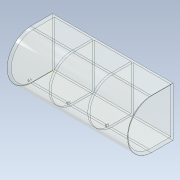
# Autodesk Inventor part: DeckelKoch_Better
Saved by Autodesk Inventor 2020 (Build 240168000, 168)
## iProperties
Created: 2022-02-02
Part Number: DeckelKoch_Better
Material: Glas
Document SubType Name: Modeling
Designer: Julian Uhl
Density: 2.18 g/cm^3
Appearance: Klar
Mass: 1224.67 g
Surface Area: 2271.98 cm^2
Volume: 561.774 cm^3
Author: Julian Uhl
Autodesk Inventor part; units mm, degrees
ref_plane "YZ Plane" through (0, 0, 0) normal (1, 0, 0) x (0, 1, 0)
ref_plane "XZ Plane" through (0, 0, 0) normal (0, 1, 0) x (-1, 0, 0)
ref_plane "XY Plane" through (0, 0, 0) normal (0, 0, 1) x (1, 0, 0)
sketch "Skizze1" plane through (0, 0, 0) normal (0, 0, 1) x (1, 0, 0)
  line L0 (-56, 0) -> (336, 0) projected
  line L1 (0, -23) -> (0, 138) projected
  line L2 (0, 0) -> (280, 0)
  line L3 (280, 0) -> (280, 115)
  line L4 (280, 115) -> (0, 115)
  line L5 (0, 115) -> (0, 0)
  line L6 (5, 5) -> (275, 5)
  line L7 (275, 5) -> (275, 110)
  line L8 (275, 110) -> (5, 110)
  line L9 (5, 110) -> (5, 5)
  dimension "d0" = 280
  dimension "d1" = 115
  dimension "d2" = 5
  dimension "d3" = 5
  dimension "d4" = 5
  dimension "d5" = 5
  constraints: 16 end point, 4 parallel, 2 horizontal, 2 perpendicular
  measures "d0" distance between parallel lines of L3 L5
  measures "d1" distance between parallel lines of L2 L4
  measures "d2" distance between parallel lines of L4 L8
  measures "d3" distance between parallel lines of L2 L6
  measures "d4" distance between parallel lines of L9 L5
  measures "d5" distance between parallel lines of L3 L7
extrude "Extrusion1" add sketch "Skizze1" along normal blind 50
sketch "Skizze3" plane through (280, 0, 0) normal (1, 0, 0) x (0, 0, -1)
  line L0 (-50, 115) -> (-50, 0) projected
  arc A0 (-50, 115) -> (-50, 0) centre (-47.5962, 57.5) ccw
  line L1 (-50, 5) -> (-50, 110) projected
  line L2 (0, 110) -> (-50, 110) projected
  arc A1 (-50, 110) -> (-50, 5) centre (-47.5962, 57.5) ccw
  point P0 (0, 0)
  dimension "d8" = 52.555
  constraints: 4 point on circle, 2 centre point, 1 coincident, 1 concentric
  measures "d8" radius of A1
extrude "Extrusion2" add sketch "Skizze3" against normal blind 275 contours L0 A1 A0
sketch "Skizze4" plane through (0, 115, 0) normal (0, 1, 0) x (1, 0, 0)
  line L0 (0, -50) -> (5, -50) projected
  line L1 (5, -50) -> (5, -105.1465) projected
  line L2 (0, -50) -> (5, -50)
  line L3 (5, -50) -> (5, -105.1465)
  line L4 (5, -105.1465) -> (0, -105.1465)
  line L5 (0, -105.1465) -> (0, -50)
  line L6 (5, -50) -> (275, -50) projected
  line L7 (280, -105.1465) -> (5, -105.1465) projected
  line L8 (275, -50) -> (280, -50)
  line L9 (280, -50) -> (280, -105.1465)
  line L10 (280, -105.1465) -> (275, -105.1465)
  line L11 (275, -105.1465) -> (275, -50)
  point P0 (0, 0)
  constraints: 16 end point, 4 parallel, 2 horizontal, 2 perpendicular, 1 point on line
extrude "Extrusion3" add sketch "Skizze4" against normal blind 115 contours L0 L1 L4 L5 | L8 L9 L7 L11
sketch "Skizze5" plane through (0, 0, 0) normal (-1, 0, 0) x (0, 0, 1)
  line L0 (50, 0) -> (105.1465, 0) projected
  arc A0 (105.1465, 57.5) -> (50, 115) centre (47.5962, 57.5) ccw projected
  line L1 (105.1465, 57.5) -> (105.1465, 0) projected
  arc A1 (50, 0) -> (50, 115) centre (47.5962, 57.5) ccw
  point P0 (0, 0)
  constraints: 3 point on circle, 1 centre point
extrude "Extrusion4" cut sketch "Skizze5" against normal blind 115
sketch "Skizze6" plane through (0, 0, 0) normal (-1, 0, 0) x (0, 0, 1)
  line L0 (105.1465, 115) -> (105.1465, 57.5) projected
  arc A0 (105.1465, 57.5) -> (50, 115) centre (47.5962, 57.5) ccw projected
  arc A1 (105.1465, 57.5) -> (50, 115) centre (47.5962, 57.5) ccw
  line L1 (50, 115) -> (105.1465, 115)
  line L2 (105.1465, 57.5) -> (105.1465, 115)
  point P0 (0, 0)
  constraints: 4 end point, 2 point on circle, 2 tangent, 1 centre point, 1 collinear, 1 horizontal
extrude "Extrusion5" cut sketch "Skizze6" against normal blind 115
sketch "Skizze7" plane through (280, 0, 0) normal (1, 0, 0) x (0, 0, -1)
  line L0 (0, 115) -> (-105.1465, 115) projected
  arc A0 (-105.1465, 57.5) -> (-50, 0) centre (-47.5962, 57.5) ccw projected
  arc A1 (-50, 115) -> (-105.1465, 57.5) centre (-47.5962, 57.5) ccw projected
  arc A2 (-52.5732, 115) -> (-50, 0) centre (-47.5081, 57.5845) ccw
  line L1 (-105.1465, 0) -> (-50, 0) projected
  line L2 (-50, 0) -> (-105.1465, 0)
  line L3 (-105.1465, 0) -> (-105.1465, 115)
  line L4 (-105.1465, 115) -> (-52.5732, 115)
  point P0 (0, 0)
  point P1 (-105.1465, 57.6691)
  constraints: 6 end point, 3 point on circle, 2 perpendicular, 1 centre point, 1 horizontal, 1 midpoint
extrude "Extrusion6" cut sketch "Skizze7" against normal blind 115
sketch "Skizze8" plane through (0, 0, 0) normal (0, 0, -1) x (-1, 0, 0)
  line L0 (-275, 5) -> (-5, 5) projected
  line L1 (-92.5, 5) -> (-92.5, 110)
  line L2 (-5, 110) -> (-275, 110) projected
  line L3 (-97.5, 5) -> (-97.5, 110)
  line L4 (-182.5, 5) -> (-182.5, 110)
  line L5 (-187.5, 5) -> (-187.5, 110)
  line L6 (0, 115) -> (0, 0) projected
  line L7 (-280, 0) -> (-280, 115) projected
  dimension "d20" = 5
  dimension "d22" = 5
  dimension "d23" = 92.5
  dimension "d24" = 92.5
  constraints: 8 end point, 8 point on line, 3 perpendicular, 1 vertical
  measures "d20" distance between parallel lines of L1 L3
  measures "d22" distance between parallel lines of L5 L4
  measures "d23" distance between parallel lines of L1 L6
  measures "d24" distance between parallel lines of L7 L5
extrude "Extrusion7" add sketch "Skizze8" against normal blind 115 contours L5 L2 L4 L0 | L3 L2 L1 L0
sketch "Skizze9" plane through (280, 0, 0) normal (1, 0, 0) x (0, 0, -1)
  arc A0 (-50, 115) -> (-50, 0) centre (-47.5962, 57.5) ccw projected
  arc A1 (-50, 115) -> (-50, 0) centre (-47.5962, 57.5) ccw
  line L0 (-50, 0) -> (-115, 0)
  line L1 (-71.1712, 5) -> (-115, 5) projected
  line L2 (-115, 0) -> (-115, 115)
  line L3 (-115, 5) -> (-115, 110) projected
  line L4 (-115, 115) -> (-50, 115)
  point P0 (0, 0)
  constraints: 6 end point, 2 point on circle, 1 centre point, 1 collinear, 1 parallel, 1 perpendicular
extrude "Extrusion8" cut sketch "Skizze9" against normal blind 280 contours A0 L1 L2 L4
sketch "Skizze10" plane through (0, 0, 0) normal (0, 0, -1) x (-1, 0, 0)
  point P0 (0, 0)
sketch "Skizze11" plane through (0, 0, 0) normal (0, 0, -1) x (-1, 0, 0)
  line L0 (0, 0) -> (-280, 0) projected
  line L1 (-92.5, 5) -> (-92.5, 110) projected
  line L2 (-97.5, 110) -> (-97.5, 5) projected
  line L3 (-187.5, 110) -> (-187.5, 5) projected
  point P0 (-50, 57.5)
  point P1 (-140, 57.5)
  point P2 (-230, 57.5)
  dimension "d29" = 57.5
  dimension "d30" = 57.5
  dimension "d31" = 57.5
  dimension "d32" = 42.5
  dimension "d33" = 42.5
  dimension "d34" = 42.5
  measures "d29" distance from line of L0 point (-50, 57.5)
  measures "d30" distance from line of L0 point (-140, 57.5)
  measures "d31" distance from line of L0 point (-230, 57.5)
  measures "d32" distance from line of point (-50, 57.5) L1
  measures "d33" distance from line of point (-140, 57.5) L2
  measures "d34" distance from line of L3 point (-230, 57.5)
hole "Bohrung1" at (50, 57.5, 0) at (140, 57.5, 0) at (230, 57.5, 0) direction (0, 0, 1) diameter 3 end through all
fillet "Rundung1" radius 0.4 3 edges at (50.0023, 56, 105.1269) (140.0023, 56, 105.1269) (230.0023, 56, 105.1269)
fillet "Rundung2" radius 0.5 6 edges at (280, 0, 25) (280, 57.5, 105.1465) (280, 115, 25) (0, 57.5, 105.1465) (0, 0, 25) (0, 115, 25)
